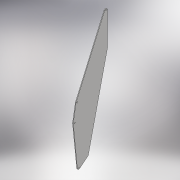
# Autodesk Inventor part: swan_plate
Saved by Autodesk Inventor 2018.2 (Build 222227000, 227)
## iProperties
Created: 2017-12-11
Part Number: swan_plate
Material: 一般
Document SubType Name: Modeling
Designer: kuwano
Density: 1 g/cm^3
Appearance: 既定
Author: kuwano
Autodesk Inventor part; units mm, degrees
ref_plane "YZ Plane" through (0, 0, 0) normal (1, 0, 0) x (0, 1, 0)
ref_plane "XZ Plane" through (0, 0, 0) normal (0, 1, 0) x (-1, 0, 0)
ref_plane "XY Plane" through (0, 0, 0) normal (0, 0, 1) x (1, 0, 0)
sketch "スケッチ1" plane through (0, 0, 0) normal (1, 0, 0) x (0, 1, 0)
  circle A0 centre (0, 0) radius 4
  circle A1 centre (30, -300) radius 4
  circle A2 centre (230, 600) radius 4
  line L0 (240, 647.8061) -> (240, -145.1416)
  line L1 (240, -145.1416) -> (21.8781, -319.2801)
  line L2 (21.8781, -319.2801) -> (-10.1864, 1.3648)
  line L3 (240, 647.8061) -> (10.3449, 122.8801)
  line L4 (10.3449, 122.8801) -> (-10.1864, 1.3648)
  circle A3 centre (20, 120) radius 4
  dimension "d0" = 30
  dimension "d1" = 300
  dimension "d2" = 8
  dimension "d3" = 8
  dimension "d4" = 600
  dimension "d5" = 230
  dimension "d6" = 8
  dimension "d9" = 10
  dimension "d11" = 10
  dimension "d13" = 10
  dimension "d14" = 10
  dimension "d16" = 10
  dimension "d17" = 10
  dimension "d18" = 10
  dimension "d19" = 8
  dimension "d20" = 120
  dimension "d21" = 20
  constraints: 10 end point, 4 centre point, 1 coincident, 1 vertical
  measures "d0" horizontal distance of A1.centre point (0, 0)
  measures "d1" vertical distance of point (0, 0) A1.centre
  measures "d2" diameter of A0
  measures "d3" diameter of A1
  measures "d4" vertical distance of point (0, 0) A2.centre
  measures "d5" horizontal distance of point (0, 0) A2.centre
  measures "d6" diameter of A2
  measures "d9" distance from line of A2.centre L0
  measures "d11" distance from line of L2 point (0, 0)
  measures "d13" distance from line of L1 A1.centre
  measures "d14" distance from line of L2 A1.centre
  measures "d16" distance from line of L3 A2.centre
  measures "d17" distance from line of L3 A3.centre
  measures "d18" distance from line of L4 A3.centre
  measures "d19" diameter of A3
  measures "d20" vertical distance of point (0, 0) A3.centre
  measures "d21" horizontal distance of A3.centre point (0, 0)
extrude "押し出し2" add sketch "スケッチ1" along normal mid plane 5
fillet "フィレット2" radius 10 4 edges at (0, 240, 647.8061) (0, 21.8781, -319.2801) (0, 10.3449, 122.8801) (0, -10.1864, 1.3648)
chamfer "面取り1" distance 500 distance2 180 1 edges at (0, 240, -145.1416) measured on face at (0, 240, -144.6416)
